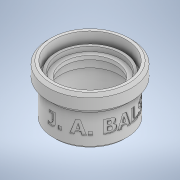
# Autodesk Inventor part: Union_Camara
Saved by Autodesk Inventor 2021 (Build 250183000, 183)
## iProperties
Created: 2021-02-05
Part Number: Union_Camara
Material: Generic
Document SubType Name: Modeling
Designer: jorge
Density: 1 g/cm^3
Appearance: Default
Author: jorge
Autodesk Inventor part; units mm, degrees
note: some values were not read from the file. Chosen so that the rebuilt part matches the saved one: direction of "Emboss1".
ref_plane "YZ Plane" through (0, 0, 0) normal (1, 0, 0) x (0, 1, 0)
ref_plane "XZ Plane" through (0, 0, 0) normal (0, 1, 0) x (-1, 0, 0)
ref_plane "XY Plane" through (0, 0, 0) normal (0, 0, 1) x (1, 0, 0)
sketch "Sketch1" plane through (0, 0, 0) normal (0, 1, 0) x (-1, 0, 0)
  circle A0 centre (0, 0) radius 16.8
  circle A1 centre (0, 0) radius 19.8
  dimension "d0" = 33.6
  dimension "d1" = 3
  constraints: 2 centre point, 1 coincident
  measures "d0" diameter of A0
  measures "d1" radial gap between concentric circles of A0 A1
extrude "Extrusion1" add sketch "Sketch1" along normal blind 20
sketch "Sketch2" plane through (0, 20, 0) normal (0, 1, 0) x (1, 0, 0)
  circle A0 centre (0, 0) radius 19.5
  circle A1 centre (0, 0) radius 22.5
  dimension "d4" = 39
  dimension "d5" = 3
  constraints: 2 centre point, 1 coincident
  measures "d4" diameter of A0
  measures "d5" radial gap between concentric circles of A0 A1
extrude "Extrusion2" add sketch "Sketch2" along normal blind 7.5
chamfer "Chamfer1" distance 2.7 angle 45 1 edges at (19.8, 20, 0)
sketch "Sketch3" plane through (0, 20, 0) normal (0, 1, 0) x (1, 0, 0)
  circle A0 centre (0, 0) radius 14
  circle A1 centre (0, 0) radius 16.8
  circle A2 centre (0, 0) radius 16.8 projected
  dimension "d11" = 28
  constraints: 2 centre point, 2 coincident, 1 concentric
  measures "d11" diameter of A0
extrude "Extrusion3" add sketch "Sketch3" against normal blind 2
sketch "Sketch4" plane through (0, 18, 0) normal (0, -1, 0) x (1, 0, 0)
  circle A0 centre (0, 0) radius 15.7
  circle A1 centre (0, 0) radius 16.8
  circle A2 centre (0, 0) radius 16.8 projected
  dimension "d14" = 31.4
  constraints: 2 centre point, 2 coincident, 1 concentric
  measures "d14" diameter of A0
extrude "Extrusion4" add sketch "Sketch4" along normal blind 5
sketch "Sketch5" plane through (0, 27.5, 0) normal (0, 1, 0) x (1, 0, 0)
  circle A0 centre (0, 0) radius 18
  circle A1 centre (0, 0) radius 19.5 projected
  circle A2 centre (0, 0) radius 16.5
  dimension "d17" = 1.5
  dimension "d18" = 3
  constraints: 2 centre point, 2 coincident
  measures "d17" radial gap between concentric circles of A1 A0
  measures "d18" radial gap between concentric circles of A2 A1
extrude "Extrusion5" add sketch "Sketch5" against normal up to surface (7.5 mm away) contours A0
chamfer "Chamfer2" distance 1.5 angle 45 1 edges at (-22.5, 27.5, 0)
sketch "Sketch6" plane through (0, 27.5, 0) normal (0, 1, 0) x (1, 0, 0)
  circle A0 centre (0, 0) radius 18
  circle A1 centre (0, 0) radius 18 projected
  constraints: 1 centre point, 1 coincident, 1 concentric
extrude "Extrusion6" cut sketch "Sketch6" against normal blind 5
chamfer "Chamfer3" distance 1.5 angle 45 1 edges at (19.8, 0, 0)
sketch "Sketch7" plane through (0, 0, 0) normal (1, 0, 0) x (0, 1, 0)
  line L0 (13.6432, 34.118) -> (13.6432, -36.6439) construction
  line L1 (13.6432, -36.6439) -> (5.5986, -36.6439) construction
  line L2 (5.5986, -36.6439) -> (5.5986, 34.118) construction
  line L3 (5.5986, 34.118) -> (13.6432, 34.118) construction
  spline S0 degree 2 poles (8.5719, 29.9373) (8.118, 29.9373) (7.3125, 30.2493) (7.0289, 30.5613) knots 0 0 0 1 2 2 2
  spline S1 degree 2 poles (7.0289, 30.5613) (6.7112, 30.913) (6.4106, 31.8716) (6.4106, 32.4956) knots 0 0 0 1 2 2 2
  spline S2 degree 2 poles (6.4106, 32.4956) (6.4106, 32.9608) (6.4787, 33.7776) (6.5467, 34.0896) knots 0 0 0 1 2 2 2
  line L4 (6.5467, 34.0896) -> (7.9649, 34.0896)
  line L5 (7.9649, 34.0896) -> (7.9649, 33.9308)
  spline S3 degree 2 poles (7.9649, 33.9308) (7.8798, 33.7209) (7.7323, 33.2614) (7.7323, 32.8984) knots 0 0 0 1 2 2 2
  spline S4 degree 2 poles (7.7323, 32.8984) (7.7323, 32.4332) (7.9932, 31.9284) (8.2315, 31.8263) knots 0 0 0 1 2 2 2
  spline S5 degree 2 poles (8.2315, 31.8263) (8.4641, 31.7185) (9.0654, 31.6958) (9.4398, 31.6958) knots 0 0 0 1 2 2 2
  line L6 (9.4398, 31.6958) -> (12.2477, 31.6958)
  line L7 (12.2477, 31.6958) -> (12.2477, 33.2955)
  line L8 (12.2477, 33.2955) -> (13.5184, 33.2955)
  line L9 (13.5184, 33.2955) -> (13.5184, 29.9373)
  line L10 (13.5184, 29.9373) -> (8.5719, 29.9373)
  line L11 (6.5184, 26.9705) -> (6.5184, 28.6326)
  line L12 (6.5184, 28.6326) -> (8.3676, 28.6326)
  line L13 (8.3676, 28.6326) -> (8.3676, 26.9705)
  line L14 (8.3676, 26.9705) -> (6.5184, 26.9705)
  line L15 (6.5184, 23.5045) -> (13.5184, 21.1391)
  line L16 (13.5184, 21.1391) -> (13.5184, 19.2217)
  line L17 (13.5184, 19.2217) -> (6.5184, 16.8562)
  line L18 (6.5184, 16.8562) -> (6.5184, 18.6658)
  line L19 (6.5184, 18.6658) -> (7.9479, 19.1026)
  line L20 (7.9479, 19.1026) -> (7.9479, 21.3036)
  line L21 (7.9479, 21.3036) -> (6.5184, 21.746)
  line L22 (6.5184, 21.746) -> (6.5184, 23.5045)
  line L23 (9.2185, 19.4883) -> (11.533, 20.2031)
  line L24 (11.533, 20.2031) -> (9.2185, 20.9235)
  line L25 (9.2185, 20.9235) -> (9.2185, 19.4883)
  line L26 (6.5184, 14.5532) -> (6.5184, 16.2152)
  line L27 (6.5184, 16.2152) -> (8.3676, 16.2152)
  line L28 (8.3676, 16.2152) -> (8.3676, 14.5532)
  line L29 (8.3676, 14.5532) -> (6.5184, 14.5532)
  spline S6 degree 2 poles (8.6626, 4.7395) (8.1407, 4.7395) (7.3522, 5.1366) (7.0913, 5.4656) knots 0 0 0 1 2 2 2
  spline S7 degree 2 poles (7.0913, 5.4656) (6.7793, 5.8627) (6.5184, 6.8044) (6.5184, 7.5361) knots 0 0 0 1 2 2 2
  line L30 (6.5184, 7.5361) -> (6.5184, 10.3327)
  line L31 (6.5184, 10.3327) -> (13.5184, 10.3327)
  line L32 (13.5184, 10.3327) -> (13.5184, 7.8651)
  spline S8 degree 2 poles (13.5184, 7.8651) (13.5184, 7.0937) (13.3992, 6.2995) (13.212, 5.9535) knots 0 0 0 1 2 2 2
  spline S9 degree 2 poles (13.212, 5.9535) (13.0135, 5.5734) (12.3328, 5.2047) (11.8903, 5.2047) knots 0 0 0 1 2 2 2
  spline S10 degree 2 poles (11.8903, 5.2047) (11.3798, 5.2047) (10.58, 5.7152) (10.3928, 6.169) knots 0 0 0 1 2 2 2
  line L33 (10.3928, 6.169) -> (10.3587, 6.169)
  spline S11 degree 2 poles (10.3587, 6.169) (10.2226, 5.5167) (9.3774, 4.7395) (8.6626, 4.7395) knots 0 0 0 1 2 2 2
  spline S12 degree 2 poles (8.691, 6.5548) (9.02, 6.5548) (9.3887, 6.8157) (9.4851, 7.0767) knots 0 0 0 1 2 2 2
  spline S13 degree 2 poles (9.4851, 7.0767) (9.5475, 7.2355) (9.5589, 7.7971) (9.5589, 8.2622) knots 0 0 0 1 2 2 2
  line L34 (9.5589, 8.2622) -> (9.5589, 8.5856)
  line L35 (9.5589, 8.5856) -> (7.7947, 8.5856)
  line L36 (7.7947, 8.5856) -> (7.7947, 8.4891)
  spline S14 degree 2 poles (7.7947, 8.4891) (7.7947, 7.8084) (7.8117, 7.2865) (7.9309, 7.0143) knots 0 0 0 1 2 2 2
  spline S15 degree 2 poles (7.9309, 7.0143) (8.0386, 6.776) (8.4357, 6.5548) (8.691, 6.5548) knots 0 0 0 1 2 2 2
  spline S16 degree 2 poles (11.5443, 6.9916) (11.7145, 6.9916) (12.0719, 7.1674) (12.1513, 7.3489) knots 0 0 0 1 2 2 2
  spline S17 degree 2 poles (12.1513, 7.3489) (12.2307, 7.5191) (12.242, 7.9956) (12.242, 8.4664) knots 0 0 0 1 2 2 2
  line L37 (12.242, 8.4664) -> (12.242, 8.5856)
  line L38 (12.242, 8.5856) -> (10.7558, 8.5856)
  line L39 (10.7558, 8.5856) -> (10.7558, 8.3643)
  spline S18 degree 2 poles (10.7558, 8.3643) (10.7558, 7.9162) (10.7728, 7.5532) (10.8636, 7.3603) knots 0 0 0 1 2 2 2
  spline S19 degree 2 poles (10.8636, 7.3603) (10.9657, 7.1504) (11.3117, 6.9916) (11.5443, 6.9916) knots 0 0 0 1 2 2 2
  line L40 (6.5184, 4.4843) -> (13.5184, 2.1188)
  line L41 (13.5184, 2.1188) -> (13.5184, 0.2015)
  line L42 (13.5184, 0.2015) -> (6.5184, -2.164)
  line L43 (6.5184, -2.164) -> (6.5184, -0.3545)
  line L44 (6.5184, -0.3545) -> (7.9479, 0.0823)
  line L45 (7.9479, 0.0823) -> (7.9479, 2.2833)
  line L46 (7.9479, 2.2833) -> (6.5184, 2.7258)
  line L47 (6.5184, 2.7258) -> (6.5184, 4.4843)
  line L48 (9.2185, 0.4681) -> (11.533, 1.1828)
  line L49 (11.533, 1.1828) -> (9.2185, 1.9032)
  line L50 (9.2185, 1.9032) -> (9.2185, 0.4681)
  line L51 (6.5184, -7.5303) -> (6.5184, -2.8618)
  line L52 (6.5184, -2.8618) -> (13.5184, -2.8618)
  line L53 (13.5184, -2.8618) -> (13.5184, -4.6203)
  line L54 (13.5184, -4.6203) -> (7.8514, -4.6203)
  line L55 (7.8514, -4.6203) -> (7.8514, -7.5303)
  line L56 (7.8514, -7.5303) -> (6.5184, -7.5303)
  spline S20 degree 2 poles (6.3936, -10.5311) (6.3936, -9.7256) (6.7056, -8.5117) (6.9325, -7.9898) knots 0 0 0 1 2 2 2
  line L57 (6.9325, -7.9898) -> (8.6002, -7.9898)
  line L58 (8.6002, -7.9898) -> (8.6002, -8.1486)
  spline S21 degree 2 poles (8.6002, -8.1486) (8.1521, -8.6762) (7.6699, -9.9412) (7.6699, -10.5368) knots 0 0 0 1 2 2 2
  spline S22 degree 2 poles (7.6699, -10.5368) (7.6699, -10.69) (7.738, -11.1835) (7.8061, -11.331) knots 0 0 0 1 2 2 2
  spline S23 degree 2 poles (7.8061, -11.331) (7.8855, -11.5125) (8.1748, -11.7678) (8.4073, -11.7678) knots 0 0 0 1 2 2 2
  spline S24 degree 2 poles (8.4073, -11.7678) (8.674, -11.7678) (9.003, -11.3537) (9.0767, -11.07) knots 0 0 0 1 2 2 2
  spline S25 degree 2 poles (9.0767, -11.07) (9.1732, -10.7126) (9.3377, -9.9015) (9.4625, -9.5441) knots 0 0 0 1 2 2 2
  spline S26 degree 2 poles (9.4625, -9.5441) (9.7461, -8.7329) (10.7161, -8.0295) (11.4422, -8.0295) knots 0 0 0 1 2 2 2
  spline S27 degree 2 poles (11.4422, -8.0295) (12.4236, -8.0295) (13.6432, -9.6916) (13.6432, -10.9396) knots 0 0 0 1 2 2 2
  spline S28 degree 2 poles (13.6432, -10.9396) (13.6432, -11.5635) (13.3879, -12.8002) (13.1723, -13.288) knots 0 0 0 1 2 2 2
  line L59 (13.1723, -13.288) -> (11.5727, -13.288)
  line L60 (11.5727, -13.288) -> (11.5727, -13.1349)
  spline S29 degree 2 poles (11.5727, -13.1349) (11.9073, -12.7434) (12.3668, -11.6203) (12.3668, -11.0303) knots 0 0 0 1 2 2 2
  spline S30 degree 2 poles (12.3668, -11.0303) (12.3668, -10.7977) (12.2988, -10.4347) (12.208, -10.2305) knots 0 0 0 1 2 2 2
  spline S31 degree 2 poles (12.208, -10.2305) (12.1343, -10.066) (11.8393, -9.8277) (11.6578, -9.8277) knots 0 0 0 1 2 2 2
  spline S32 degree 2 poles (11.6578, -9.8277) (11.3855, -9.8277) (11.0735, -10.2078) (10.9487, -10.7524) knots 0 0 0 1 2 2 2
  spline S33 degree 2 poles (10.9487, -10.7524) (10.8693, -11.1041) (10.7161, -11.7564) (10.5856, -12.1308) knots 0 0 0 1 2 2 2
  spline S34 degree 2 poles (10.5856, -12.1308) (10.319, -12.8569) (9.4341, -13.566) (8.708, -13.566) knots 0 0 0 1 2 2 2
  spline S35 degree 2 poles (8.708, -13.566) (7.6642, -13.566) (6.3936, -11.9266) (6.3936, -10.5311) knots 0 0 0 1 2 2 2
  line L61 (6.5184, -14.4679) -> (13.5184, -14.4679)
  line L62 (13.5184, -14.4679) -> (13.5184, -19.1989)
  line L63 (13.5184, -19.1989) -> (12.1853, -19.1989)
  line L64 (12.1853, -19.1989) -> (12.1853, -16.2151)
  line L65 (12.1853, -16.2151) -> (10.9544, -16.2151)
  line L66 (10.9544, -16.2151) -> (10.9544, -18.9663)
  line L67 (10.9544, -18.9663) -> (9.6213, -18.9663)
  line L68 (9.6213, -18.9663) -> (9.6213, -16.2151)
  line L69 (9.6213, -16.2151) -> (7.8514, -16.2151)
  line L70 (7.8514, -16.2151) -> (7.8514, -19.1989)
  line L71 (7.8514, -19.1989) -> (6.5184, -19.1989)
  line L72 (6.5184, -19.1989) -> (6.5184, -14.4679)
  line L73 (6.5184, -25.0587) -> (6.5184, -20.3901)
  line L74 (6.5184, -20.3901) -> (13.5184, -20.3901)
  line L75 (13.5184, -20.3901) -> (13.5184, -22.1486)
  line L76 (13.5184, -22.1486) -> (7.8514, -22.1486)
  line L77 (7.8514, -22.1486) -> (7.8514, -25.0587)
  line L78 (7.8514, -25.0587) -> (6.5184, -25.0587)
  line L79 (6.5184, -30.5668) -> (6.5184, -25.8982)
  line L80 (6.5184, -25.8982) -> (13.5184, -25.8982)
  line L81 (13.5184, -25.8982) -> (13.5184, -27.6567)
  line L82 (13.5184, -27.6567) -> (7.8514, -27.6567)
  line L83 (7.8514, -27.6567) -> (7.8514, -30.5668)
  line L84 (7.8514, -30.5668) -> (6.5184, -30.5668)
  spline S36 degree 2 poles (6.3936, -33.5676) (6.3936, -32.7621) (6.7056, -31.5481) (6.9325, -31.0263) knots 0 0 0 1 2 2 2
  line L85 (6.9325, -31.0263) -> (8.6002, -31.0263)
  line L86 (8.6002, -31.0263) -> (8.6002, -31.1851)
  spline S37 degree 2 poles (8.6002, -31.1851) (8.1521, -31.7126) (7.6699, -32.9776) (7.6699, -33.5733) knots 0 0 0 1 2 2 2
  spline S38 degree 2 poles (7.6699, -33.5733) (7.6699, -33.7264) (7.738, -34.2199) (7.8061, -34.3674) knots 0 0 0 1 2 2 2
  spline S39 degree 2 poles (7.8061, -34.3674) (7.8855, -34.549) (8.1748, -34.8042) (8.4073, -34.8042) knots 0 0 0 1 2 2 2
  spline S40 degree 2 poles (8.4073, -34.8042) (8.674, -34.8042) (9.003, -34.3901) (9.0767, -34.1065) knots 0 0 0 1 2 2 2
  spline S41 degree 2 poles (9.0767, -34.1065) (9.1732, -33.7491) (9.3377, -32.9379) (9.4625, -32.5806) knots 0 0 0 1 2 2 2
  spline S42 degree 2 poles (9.4625, -32.5806) (9.7461, -31.7694) (10.7161, -31.066) (11.4422, -31.066) knots 0 0 0 1 2 2 2
  spline S43 degree 2 poles (11.4422, -31.066) (12.4236, -31.066) (13.6432, -32.728) (13.6432, -33.976) knots 0 0 0 1 2 2 2
  spline S44 degree 2 poles (13.6432, -33.976) (13.6432, -34.6) (13.3879, -35.8366) (13.1723, -36.3245) knots 0 0 0 1 2 2 2
  line L87 (13.1723, -36.3245) -> (11.5727, -36.3245)
  line L88 (11.5727, -36.3245) -> (11.5727, -36.1713)
  spline S45 degree 2 poles (11.5727, -36.1713) (11.9073, -35.7799) (12.3668, -34.6567) (12.3668, -34.0668) knots 0 0 0 1 2 2 2
  spline S46 degree 2 poles (12.3668, -34.0668) (12.3668, -33.8342) (12.2988, -33.4712) (12.208, -33.2669) knots 0 0 0 1 2 2 2
  spline S47 degree 2 poles (12.208, -33.2669) (12.1343, -33.1024) (11.8393, -32.8642) (11.6578, -32.8642) knots 0 0 0 1 2 2 2
  spline S48 degree 2 poles (11.6578, -32.8642) (11.3855, -32.8642) (11.0735, -33.2443) (10.9487, -33.7888) knots 0 0 0 1 2 2 2
  spline S49 degree 2 poles (10.9487, -33.7888) (10.8693, -34.1405) (10.7161, -34.7929) (10.5856, -35.1673) knots 0 0 0 1 2 2 2
  spline S50 degree 2 poles (10.5856, -35.1673) (10.319, -35.8934) (9.4341, -36.6024) (8.708, -36.6024) knots 0 0 0 1 2 2 2
  spline S51 degree 2 poles (8.708, -36.6024) (7.6642, -36.6024) (6.3936, -34.9631) (6.3936, -33.5676) knots 0 0 0 1 2 2 2
  point P0 (0, 0)
  constraints: 2 other
emboss "Emboss1" sketch "Sketch7" operation cut depth 0.5 direction (-1, 0, 0) wrap yes faces at (-19.7358, 12.0334, -1.5932)
body "Solid1"
